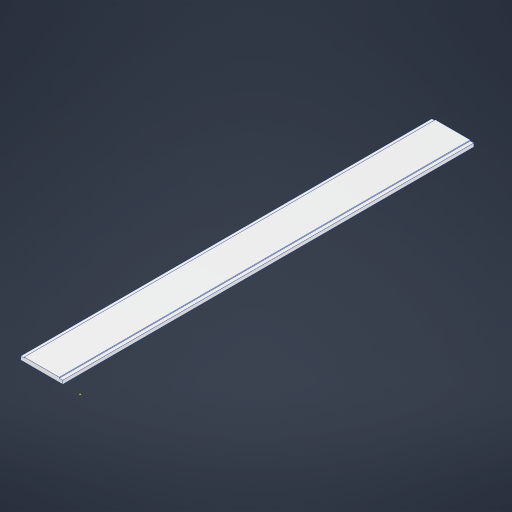
# Autodesk Inventor part: TopZakrivka
Saved by Autodesk Inventor 2024 (Build 280153000, 153)
## iProperties
Created: 2023-12-21
Part Number: TopZakrivka
Material: Aluminum 6061
Document SubType Name: Modeling
Designer: KirikDK
Mass: 2355.26 g
Surface Area: 2011.36 cm^2
Volume: 872.32 cm^3
Density: 2.7 g/cm^3
Appearance: Aluminum - Flat
Author: KirikDK
Autodesk Inventor part; units mm, degrees
ref_plane "YZ Plane" through (0, 0, 0) normal (1, 0, 0) x (0, 1, 0)
ref_plane "XZ Plane" through (0, 0, 0) normal (0, 1, 0) x (-1, 0, 0)
ref_plane "XY Plane" through (0, 0, 0) normal (0, 0, 1) x (1, 0, 0)
sketch "Sketch1" plane through (0, 0, 0) normal (0, 1, 0) x (-1, 0, 0)
  line L0 (135.7143, 497.619) -> (39.7143, 497.619)
  line L1 (39.7143, 497.619) -> (39.7143, -442.381)
  line L2 (39.7143, -442.381) -> (135.7143, -442.381)
  line L3 (135.7143, -442.381) -> (135.7143, 497.619)
  point P0 (0, 0)
  dimension "d0" = 940
  dimension "d1" = 96
  constraints: 8 end point, 2 parallel, 1 horizontal, 1 perpendicular
  measures "d0" distance of L2.end L0.start
  measures "d1" distance of L0.start L0.end
extrude "Extrusion1" add sketch "Sketch1" along normal blind 14
sketch "Sketch2" plane through (-135.7143, 0, 497.619) normal (0, 0, 1) x (1, 0, 0)
  point P0 (135.7143, 0)
sketch "Sketch3" plane through (-135.7143, 0, 497.619) normal (0, 0, 1) x (1, 0, 0)
  line L0 (96, 14) -> (0, 14) projected
  line L1 (0, 14) -> (8, 14)
  line L2 (8, 14) -> (8, 8)
  line L3 (8, 8) -> (0, 8)
  line L4 (0, 8) -> (0, 14)
  line L5 (96, 14) -> (88, 14)
  line L6 (88, 14) -> (88, 8)
  line L7 (88, 8) -> (96, 8)
  line L8 (96, 8) -> (96, 14)
  line L9 (8, 14) -> (88, 14)
  line L10 (88, 14) -> (88, 10)
  line L11 (88, 10) -> (8, 10)
  line L12 (8, 10) -> (8, 14)
  point P0 (135.7143, 0)
  point P1 (8, 10)
  dimension "d4" = 8
  dimension "d5" = 6
  dimension "d6" = 6
  constraints: 24 end point, 6 parallel, 3 horizontal, 3 perpendicular, 1 point on line
  measures "d4" distance of L2.end L3.end
  measures "d5" distance of L1.end L2.end
  measures "d6" distance of L5.end L6.end
extrude "Extrusion2" cut sketch "Sketch3" against normal through all
body "Solid1"
